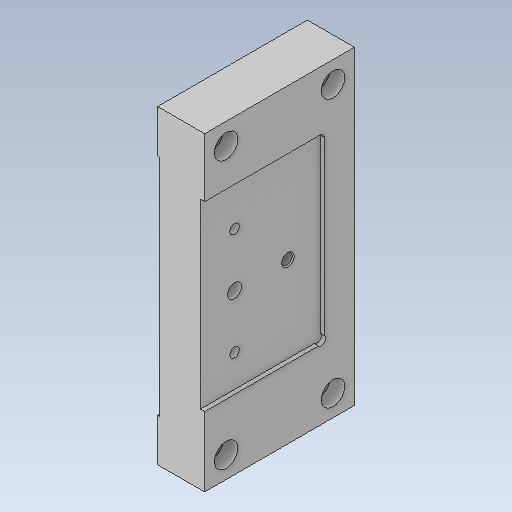
# Autodesk Inventor part: FAB-OX0009
Saved by Autodesk Inventor 2020 (Build 240168000, 168)
## iProperties
Created: 2017-01-19
Part Number: FAB-OX0009
Material: Generic
Document SubType Name: Modeling
Designer: map
Density: 1 g/cm^3
Appearance: Default
Description: Overview Flip Mirror Mount
Author: map
Revision Number: 01
Autodesk Inventor part; units mm, degrees
ref_plane "YZ Plane" through (0, 0, 0) normal (1, 0, 0) x (0, 1, 0)
ref_plane "XZ Plane" through (0, 0, 0) normal (0, 1, 0) x (-1, 0, 0)
ref_plane "XY Plane" through (0, 0, 0) normal (0, 0, 1) x (1, 0, 0)
sketch "Sketch1" plane through (0, 0, 0) normal (1, 0, 0) x (0, 1, 0)
  line L0 (0, 0) -> (-145, 0)
  line L1 (-145, 0) -> (-145, -70)
  line L2 (-145, -70) -> (0, -70)
  line L3 (0, -70) -> (0, 0)
  dimension "d0" = 145
  dimension "d1" = 70
  constraints: 8 end point, 2 parallel, 1 coincident, 1 horizontal, 1 perpendicular
  measures "d0" distance of L2.end L1.end
  measures "d1" distance of L1.end L0.end
extrude "Extrusion1" add sketch "Sketch1" along normal blind 20
sketch "Sketch5" plane through (20, 0, 0) normal (1, 0, 0) x (0, 0, -1)
  line L0 (49.9481, -33) -> (-5.5519, -33) projected
  arc A0 (-6.6519, -32.6703) -> (-5.5519, -33) centre (-5.5519, -31) ccw projected
  line L1 (-6.6519, -32.6703) -> (-6.6519, -47) projected
  arc A1 (-9.5519, -49.9) -> (-6.6519, -47) centre (-9.5519, -47) ccw projected
  line L2 (-9.5519, -49.9) -> (-23.8816, -49.9) projected
  arc A2 (-23.5519, -51) -> (-23.8816, -49.9) centre (-25.5519, -51) ccw projected
  line L3 (-23.5519, -51) -> (-23.5519, -106.5) projected
  arc A3 (-23.5519, -106.5) -> (-18.0519, -112) centre (-18.0519, -106.5) ccw projected
  line L4 (-18.0519, -112) -> (49.9481, -112) projected
  arc A4 (49.9481, -112) -> (55.4481, -106.5) centre (49.9481, -106.5) ccw projected
  line L5 (55.4481, -106.5) -> (55.4481, -38.5) projected
  arc A5 (55.4481, -38.5) -> (49.9481, -33) centre (49.9481, -38.5) ccw projected
  circle A6 centre (15.9481, -97.5) radius 1.65 projected
  circle A7 centre (15.9481, -47.5) radius 1.65 projected
  circle A8 centre (50.6979, -96.4808) radius 0.6924 projected
  circle A9 centre (-9.0519, -72.5) radius 5.5 projected
  circle A10 centre (40.9481, -72.5) radius 5.5 projected
  circle A11 centre (15.9481, -72.5) radius 2.5 projected
  circle A12 centre (-9.0519, -97.5) radius 4 projected
  circle A13 centre (40.9481, -47.5) radius 4 projected
  circle A14 centre (28.9481, -89.75) radius 1.5 projected
  circle A15 centre (47.9481, -43.6) radius 1.5 projected
  circle A16 centre (-12.9519, -104.5) radius 1.5 projected
  circle A17 centre (33.1981, -85.5) radius 1.5 projected
  circle A18 centre (-1.8019, -49.6) radius 1.5 projected
  circle A19 centre (-6.9519, -54.75) radius 1.5 projected
  line L6 (43.2888, -99.6225) -> (54.231, -96.5) projected
  line L7 (54.231, -96.5) -> (50.8902, -107.3775) projected
  line L8 (50.8902, -107.3775) -> (39.9481, -110.5) projected
  line L9 (39.9481, -110.5) -> (43.2888, -99.6225) projected
  line L10 (49.9481, -32.5) -> (-5.5519, -32.5) projected
  arc A20 (55.9481, -38.5) -> (49.9481, -32.5) centre (49.9481, -38.5) ccw projected
  line L11 (55.9481, -106.5) -> (55.9481, -38.5) projected
  arc A21 (49.9481, -112.5) -> (55.9481, -106.5) centre (49.9481, -106.5) ccw projected
  line L12 (-18.0519, -112.5) -> (49.9481, -112.5) projected
sketch "Sketch10" plane through (20, 0, 0) normal (1, 0, 0) x (0, 0, -1)
  line L0 (0, 0) -> (0, -145) construction
  line L1 (0, -145) -> (70, -145) construction
  line L2 (70, -145) -> (70, 0) construction
  line L3 (70, 0) -> (0, 0) construction
  line L4 (49.9481, -32.5) -> (-5.5519, -32.5) construction
  line L5 (55.9481, -106.5) -> (55.9481, -38.5) construction
  line L6 (-18.0519, -112.5) -> (49.9481, -112.5) construction
  line L7 (0, 0) -> (0, -145) construction
  line L8 (0, -112.5) -> (0, -145)
  line L9 (0, -145) -> (70, -145) projected
  line L10 (0, -145) -> (70, -145)
  line L11 (70, -145) -> (70, 0) projected
  line L12 (70, -145) -> (70, 0)
  line L13 (70, 0) -> (0, 0) projected
  line L14 (70, 0) -> (0, 0)
  line L15 (0, 0) -> (0, -27.5)
  line L16 (0, -27.5) -> (53.9481, -27.5)
  line L17 (55.9481, -29.5) -> (55.9481, -109.6716)
  line L18 (53.1196, -112.5) -> (0, -112.5)
  arc A0 (55.9481, -29.5) -> (53.9481, -27.5) centre (53.9481, -29.5) ccw
  line L19 (53.1196, -112.5) -> (55.9481, -109.6716) construction
  arc A1 (53.1196, -112.5) -> (55.9481, -109.6716) centre (54.5339, -111.0858) ccw
  dimension "d74" = 85
  dimension "d76" = 2
  dimension "d79" = 45
  dimension "d80" = 4
  constraints: 18 end point, 6 collinear, 4 point on circle, 3 point on line, 2 centre point, 2 tangent, 1 horizontal, 1 midpoint, 1 perpendicular
  measures "d74" distance between parallel lines of L16 L6
  measures "d76" radius of A0
  measures "d79" angle of L19 L18
  measures "d80" distance of L18.start L17.end
extrude "Extrusion2" add sketch "Sketch10" along normal blind 2
sketch "Sketch2" plane through (22, 0, 0) normal (1, 0, 0) x (0, 0, -1)
  line L0 (-23.2163, -0.5426) -> (-23.2163, -85.5426) construction
  line L1 (10, -10) -> (60, -10) construction
  line L2 (60, -10) -> (60, -135) construction
  line L3 (60, -135) -> (10, -135) construction
  line L4 (10, -135) -> (10, -10) construction
  line L5 (-23.2163, -85.5426) -> (29.9034, -85.5426)
  arc A0 (29.9034, -85.5426) -> (32.7318, -82.7142) centre (31.3176, -84.1284) ccw
  line L6 (32.7318, -82.7142) -> (32.7318, -2.5426)
  arc A1 (32.7318, -2.5426) -> (30.7318, -0.5426) centre (30.7318, -2.5426) ccw
  line L7 (30.7318, -0.5426) -> (-23.2163, -0.5426)
  line L8 (70, 0) -> (0, 0) projected
  line L9 (70, -145) -> (70, 0) projected
  dimension "d4" = 50
  dimension "d5" = 125
  dimension "d81" = 10
  dimension "d82" = 10
  constraints: 16 end point, 4 coincident, 4 point on circle, 2 centre point, 2 parallel, 1 horizontal, 1 perpendicular
  measures "d4" distance of L2.end L3.end
  measures "d5" distance of L1.end L2.end
  measures "d81" distance between parallel lines of L8 L1
  measures "d82" distance between parallel lines of L9 L2
hole "M6CBoreToTable" at (22, -10, -10) at (22, -10, -60) at (22, -135, -60) at (22, -135, -10) direction (-1, 0, 0) diameter 6.6 end through all counterbore diameter 11 counterbore depth 6.8 clearance for "Socket Head Cap Screw ISO 4762" size "M6" standard "ISO"
hole "Hole9" at (20, -72.5, -40.9481) direction (-1, 0, 0) diameter 4.917 depth 17.1 tip angle 118 thread size "M6x1" class "6H" standard "ISO Metric profile"
chamfer "Chamfer1" distance 0.5 angle 45 1 edges at (20, -72.5, -38.4896)
sketch "Sketch11" plane through (0, 0, 0) normal (-1, 0, 0) x (0, 0, 1)
  circle A0 centre (-60, -10) radius 3.3 construction
  circle A1 centre (-10, -135) radius 3.3 construction
  line L0 (-60, -10) -> (-10, -10) construction
  line L1 (-10, -10) -> (-10, -135) construction
  line L2 (-10, -135) -> (-60, -135) construction
  line L3 (-60, -135) -> (-60, -10) construction
  circle A2 centre (-35, -10) radius 2
  line L4 (-35, -138) -> (-35, -132) construction
  line L5 (-33, -138) -> (-33, -132)
  line L6 (-37, -132) -> (-37, -138)
  arc A3 (-37, -138) -> (-33, -138) centre (-35, -138) ccw
  arc A4 (-33, -132) -> (-37, -132) centre (-35, -132) ccw
  point P0 (0, 0)
  point P1 (-35, -135)
  dimension "d86" = 4
  dimension "d87" = 3
  dimension "d88" = 4
  constraints: 16 end point, 4 point on circle, 4 tangent, 3 centre point, 3 coincident, 3 midpoint, 3 parallel, 2 perpendicular, 1 horizontal
  measures "d86" diameter of A2
  measures "d87" distance of point (-35, -135) L4.end
  measures "d88" diameter of A4
hole "Hole10" at (0, -10, -35) at (0, -135, -35) at (0, -132, -35) at (0, -138, -35) direction (1, 0, 0) diameter 4 depth 10
extrude "Extrusion3" cut sketch "Sketch11" against normal up to surface (10 mm away) contours A3 L6 A4 L5
sketch "Sketch12" plane through (0, 0, 0) normal (-1, 0, 0) x (0, 0, 1)
  line L0 (-70, -145) -> (-70, 0) projected
  line L1 (0, -112.5) -> (0, -145) projected
  line L2 (-70, -20) -> (0, -20)
  line L3 (0, -20) -> (0, -125)
  line L4 (0, -125) -> (-70, -125)
  line L5 (-70, -125) -> (-70, -20)
  line L6 (-70, 0) -> (0, 0) projected
  line L7 (0, -145) -> (-70, -145) projected
  dimension "d98" = 20
  dimension "d99" = 20
  constraints: 8 end point, 2 parallel, 2 point on line, 1 horizontal, 1 perpendicular
  measures "d98" distance between parallel lines of L6 L2
  measures "d99" distance between parallel lines of L4 L7
extrude "Extrusion4" cut sketch "Sketch12" against normal blind 1 contours L0 L2 L3 L1 L4
sketch "Sketch6" plane through (1, 0, 0) normal (-1, 0, 0) x (0, 0, 1)
  point P0 (0, 0)
  point P1 (-15.9481, -47.5)
  point P2 (-15.9481, -97.5)
sketch "Sketch8" plane through (1, 0, 0) normal (-1, 0, 0) x (0, 0, 1)
  circle A0 centre (-15.9481, -72.5) radius 2.5
  point P0 (0, 0)
  constraints: 1 centre point
hole "M6CBoreToMounted" at (1, -72.5, -15.9481) direction (1, 0, 0) diameter 6.6 end through all counterbore diameter 11 counterbore depth 6.8 clearance for "Socket Head Cap Screw ISO 4762" size "M6" standard "ISO"
hole "Hole8" at (1, -47.5, -15.9481) at (1, -97.5, -15.9481) direction (1, 0, 0) diameter 4.5 end through all counterbore diameter 8 counterbore depth 10 clearance for "Socket Head Cap Screw ISO 4762" size "M4" standard "ISO"
equation "\"d86\" = d88"
equation "\"d89\" = d88"
body "Solid1"
